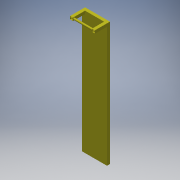
# Autodesk Inventor part: rung
Saved by Autodesk Inventor 2017 SP1 (Build 210196100, 196)
## iProperties
Created: 2018-03-18
Part Number: rung
Material: Aluminum 6061
Document SubType Name: Modeling
Designer: Ben
Density: 2.7 g/cm^3
Appearance: Canary
Author: Ben
Autodesk Inventor part; units mm, degrees
ref_plane "YZ Plane" through (0, 0, 0) normal (1, 0, 0) x (0, 1, 0)
ref_plane "XZ Plane" through (0, 0, 0) normal (0, 1, 0) x (-1, 0, 0)
ref_plane "XY Plane" through (0, 0, 0) normal (0, 0, 1) x (1, 0, 0)
sketch "Sketch1" plane through (0, 0, 0) normal (0, 0, 1) x (1, 0, 0)
  line L0 (-165.1, 0) -> (165.1, 0) construction
  line L1 (-215.9, -25.4) -> (-165.1, -25.4)
  line L2 (-165.1, -25.4) -> (-165.1, 25.4)
  line L3 (-165.1, 25.4) -> (-215.9, 25.4)
  line L4 (-215.9, 25.4) -> (-215.9, -25.4)
  line L5 (-215.9, -25.4) -> (-165.1, 25.4) construction
  line L6 (-165.1, -25.4) -> (-215.9, 25.4) construction
  line L7 (215.9, -25.4) -> (165.1, -25.4)
  line L8 (165.1, -25.4) -> (165.1, 25.4)
  line L9 (165.1, 25.4) -> (215.9, 25.4)
  line L10 (215.9, 25.4) -> (215.9, -25.4)
  line L11 (215.9, -25.4) -> (165.1, 25.4) construction
  line L12 (165.1, -25.4) -> (215.9, 25.4) construction
  line L13 (-168.275, 22.225) -> (-168.275, -22.225)
  line L14 (-168.275, -22.225) -> (-212.725, -22.225)
  line L15 (-212.725, -22.225) -> (-212.725, 22.225)
  line L16 (-212.725, 22.225) -> (-168.275, 22.225)
  line L17 (212.725, -22.225) -> (168.275, -22.225)
  line L18 (168.275, -22.225) -> (168.275, 22.225)
  line L19 (168.275, 22.225) -> (212.725, 22.225)
  line L20 (212.725, 22.225) -> (212.725, -22.225)
  point P0 (0, 0)
  point P1 (0, 0)
  point P2 (-190.5, 0)
  point P3 (190.5, 0)
  dimension "d0" = 330.2
  dimension "d1" = 50.8
  dimension "d2" = 3.175
  dimension "d3" = 3.175
  constraints: 42 end point, 8 parallel, 7 midpoint, 4 perpendicular, 3 equal length, 3 horizontal, 1 coincident, 6 other
  measures "d0" distance of L0.start L0.end
  measures "d1" distance of L2.end L3.end
  measures "d2" distance between parallel lines of L2 L13
  measures "d3" distance between parallel lines of L10 L20
extrude "Extrusion1" add sketch "Sketch1" along normal blind 209.55
sketch "Sketch2" plane through (215.9, -25.4, 0) normal (1, 0, 0) x (0, 0, -1)
  line L0 (0, 25.4) -> (-209.55, 25.4) construction
  line L1 (-209.55, 3.175) -> (-209.55, 47.625) construction
  circle A0 centre (-190.5, 25.4) radius 15.875
  circle A1 centre (-190.5, 25.4) radius 12.7
  dimension "d6" = 31.75
  dimension "d7" = 19.05
  dimension "d8" = 3.175
  constraints: 2 centre point, 2 end point, 1 midpoint, 1 point on line
  measures "d6" diameter of A0
  measures "d7" distance from line of L1 A0.centre
  measures "d8" radial gap between concentric circles of A0 A1
extrude "Extrusion2" add sketch "Sketch2" against normal up to surface (431.8 mm away)
sketch "Sketch3" plane through (-215.9, 25.4, 0) normal (0, 1, 0) x (1, 0, 0)
  line L0 (431.8, 0) -> (0, 0)
  line L1 (0, 0) -> (0, 50.8)
  line L2 (0, 50.8) -> (431.8, 50.8)
  line L3 (431.8, 50.8) -> (431.8, 0)
  point P0 (215.9, 0)
  point P1 (215.9, 0)
  dimension "d11" = 431.8
  dimension "d12" = 50.8
  constraints: 8 end point, 2 parallel, 1 coincident, 1 horizontal, 1 midpoint, 1 perpendicular
  measures "d11" distance of L1.end L2.end
  measures "d12" distance of L0.end L1.end
extrude "Extrusion3" add sketch "Sketch3" against normal blind 2143.125
body "Solid1"
